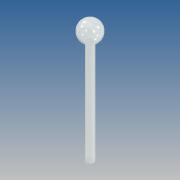
# Autodesk Inventor part: 3104_Example Bulb_V1
Saved by Autodesk Inventor 2020 (Build 240168000, 168)
## iProperties
Created: 2019-11-12
Part Number: 3104_Example Bulb_V1
Material: Glass
Document SubType Name: Modeling
Designer: RFLab
Density: 2.18 g/cm^3
Appearance: Clear
Author: RFLab
Autodesk Inventor part; units mm, degrees
ref_plane "YZ Plane" through (0, 0, 0) normal (1, 0, 0) x (0, 1, 0)
ref_plane "XZ Plane" through (0, 0, 0) normal (0, 1, 0) x (-1, 0, 0)
ref_plane "XY Plane" through (0, 0, 0) normal (0, 0, 1) x (1, 0, 0)
sketch "Sketch1" plane through (0, 0, 0) normal (0, 0, 1) x (1, 0, 0)
  line L0 (0, 0) -> (0, 23) construction
  line L1 (0.75, 0) -> (0.75, 21.0385)
  arc A0 (0.75, 21.0385) -> (0, 25.1) centre (0, 23) ccw
  arc A1 (0, 21.1) -> (0, 24.9) centre (0, 23) ccw
  line L2 (0, 8.5) -> (0, 25.1)
  line L3 (0.6, 0) -> (0.6, 21.1972)
  line L4 (0.6, 0) -> (0.75, 0)
  point P0 (0.75, 21.4189)
  dimension "d0" = 4.2
  dimension "d1" = 3.8
  dimension "d2" = 23
  dimension "d3" = 0.75
  dimension "d4" = 0.15
  constraints: 10 end point, 5 point on circle, 3 point on line, 2 centre point, 2 coincident, 2 parallel, 2 vertical, 1 horizontal, 1 horizontal alignment
  measures "d0" diameter of A0
  measures "d1" diameter of A1
  measures "d2" distance of L0.start L0.end
  measures "d3" distance between parallel lines of L0 L1
  measures "d4" distance between parallel lines of L1 L3
revolve "Revolution1" add sketch "Sketch1" angle 360 about axis through (0, 0, 0) along (0, 1, 0) contours L4 L3 A1 L2 A0 L1
sketch "Sketch2" plane through (0, 0, 0) normal (0, 0, 1) x (1, 0, 0)
  arc A0 (0.6, 21.1972) -> (-0.6, 21.1972) centre (0, 23) ccw projected
  line L0 (0.6, 0) -> (0.6, 21.1972) projected
  circle A1 centre (0, 23) radius 1.9
  line L1 (-0.6, 0) -> (-0.6, 21.1972) projected
  line L2 (0.6, 21.1972) -> (-0.6, 21.1972)
  line L3 (-0.6, 21.1972) -> (-0.6, 19.6972)
  line L4 (-0.6, 19.6972) -> (0.6, 19.6972)
  line L5 (0.6, 19.6972) -> (0.6, 21.1972)
  line L6 (0, 23) -> (0, 19.6972)
  line L7 (0, 21.1) -> (0, 19.6972)
  point P0 (0, 0)
  point P1 (0, 21.1)
  dimension "d6" = 1.5
  constraints: 12 end point, 2 parallel, 1 coincident, 1 horizontal, 1 midpoint, 1 perpendicular, 1 point on circle, 1 point on line, 1 vertical, 1 vertical alignment, 3 other
  measures "d6" distance of L3.end L2.end
revolve "Revolution2" [suppressed]
body "Solid1"
body "Solid2"
